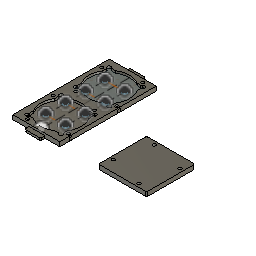
CoasterCutHolder_Double (Autodesk Fusion 360 design; units mm, degrees)
Autodesk Fusion 360 part; units mm, degrees
sketch "Sketch1" plane through (0, 0, 0) normal (0, 0, 1) x (1, 0, 0)
  line L0 (0, 0) -> (110, 0)
  line L1 (110, 0) -> (110, 110)
  line L2 (110, 110) -> (0, 110)
  line L3 (0, 110) -> (0, 0)
  line L4 (152.6101, 110) -> (152.6101, -10) construction
  line L5 (305.2202, 110) -> (305.2202, 0)
  line L6 (305.2202, 0) -> (195.2202, 0)
  line L7 (195.2202, 0) -> (195.2202, 110)
  line L8 (195.2202, 110) -> (305.2202, 110)
  line L9 (211.6202, 93.6) -> (288.8202, 93.6) construction
  line L10 (288.8202, 93.6) -> (288.8202, 16.4) construction
  line L11 (288.8202, 16.4) -> (211.6202, 16.4) construction
  line L12 (211.6202, 16.4) -> (211.6202, 93.6) construction
  line L13 (260, 93.6) -> (260, 110) construction
  line L14 (258.2734, 16.4) -> (258.2734, 0) construction
  line L15 (288.8202, 57.8839) -> (305.2202, 57.8839) construction
  line L16 (211.6202, 57.8839) -> (195.2202, 57.8839) construction
  line L17 (250.2202, 93.6) -> (250.2202, 110) construction
  line L18 (288.8202, 55) -> (305.2202, 55) construction
  line L19 (250.2202, 16.4) -> (250.2202, 0) construction
  line L20 (211.6202, 55) -> (195.2202, 55) construction
  line L21 (110, 67.7) -> (110, 42.3)
  line L22 (0, 42.3) -> (0, 67.7)
  line L23 (-12.7, 55) -> (0, 55) construction
  line L24 (0, 55) -> (110, 55) construction
  line L25 (122.7, 55) -> (110, 55) construction
  point P0 (250.2202, 8.2)
  point P1 (297.0202, 55)
  point P2 (250.2202, 101.8)
  point P3 (203.4202, 55)
  dimension "d3" = 110
  dimension "d4" = 110
  dimension "d17" = 77.2
  constraint horizontal L0
  constraint vertical L1
  constraint horizontal L2
  constraint vertical L3
  constraint coincident L0.start L3.end
  constraint vertical L4
  constraint symmetric L0.start L4 L5.end
  constraint symmetric L0.end L4 L6.end
  constraint symmetric L1.end L4 L7.end
  constraint symmetric L2.end L4 L5.start
  constraint horizontal L9
  constraint vertical L10
  constraint horizontal L11
  constraint vertical L12
  constraint coincident L9 L13.start
  constraint coincident L8 L13.end
  constraint perpendicular L8 L13
  constraint coincident L11 L14.start
  constraint coincident L6 L14.end
  constraint perpendicular L6 L14
  constraint coincident L10 L15.start
  constraint coincident L5 L15.end
  constraint perpendicular L5 L15
  constraint coincident L12 L16.start
  constraint coincident L7 L16.end
  constraint perpendicular L7 L16
  constraint equal L15 L16
  constraint equal L13 L15
  constraint equal L13 L14
  constraint midpoint L9 L17.start
  constraint midpoint L8 L17.end
  constraint midpoint L10 L18.start
  constraint midpoint L5 L18.end
  constraint midpoint L11 L19.start
  constraint midpoint L6 L19.end
  constraint midpoint L12 L20.start
  constraint midpoint L7 L20.end
  constraint midpoint L19 P0
  constraint midpoint L18 P1
  constraint midpoint L17 P2
  constraint midpoint L20 P3
  constraint vertical L21
  constraint coincident L1 L21.end
  constraint vertical L22
  constraint coincident L3 L22.end
  constraint midpoint L22 L23.end
  constraint midpoint L3 L23.end
  constraint midpoint L1 L24.end
  constraint midpoint L21 L24.end
  constraint collinear L23 L24
  measures "d3" distance of L0.start L2.end
  measures "d4" distance of L0.start L0.end
  measures "d17" distance of L9.start L9.end
extrude "Extrude1" add sketch "Sketch1" along normal blind 10 contours L0 L1 L2 L3 L21 L22 makes body 1
sketch "Sketch2" plane through (0, 0, 10) normal (0, 0, 1) x (-1, 0, 0)
  line L0 (0, -110) -> (0, 0)
  line L1 (0, 0) -> (-110, 0)
  line L2 (-110, 0) -> (-110, -110)
  line L3 (-110, -110) -> (0, -110)
  line L4 (-16.4, -93.6) -> (-93.6, -93.6)
  line L5 (-93.6, -93.6) -> (-93.6, -16.4)
  line L6 (-93.6, -16.4) -> (-16.4, -16.4)
  line L7 (-16.4, -16.4) -> (-16.4, -93.6)
  line L8 (0, -65.0851) -> (-16.4, -65.0851) construction
  line L9 (-93.6, -65.0851) -> (-110, -65.0851) construction
  line L10 (-60.9171, -93.6) -> (-60.9171, -110) construction
  line L11 (-67.2958, -16.4) -> (-67.2958, 0) construction
  circle A0 centre (-16.4, -93.6) radius 4
  circle A1 centre (-93.6, -93.6) radius 4
  circle A2 centre (-93.6, -16.4) radius 4
  circle A3 centre (-16.4, -16.4) radius 4
  line L12 (0, -84.4385) -> (-16.4, -84.0438) construction
  line L13 (-25.6464, -16.4) -> (-25.6464, 0) construction
  line L14 (-93.6, -25.6464) -> (-110, -25.6464) construction
  line L15 (-84.3536, -93.6) -> (-84.3536, -110) construction
  line L16 (-110, -110) -> (0, -110)
  line L17 (-110, 0) -> (-110, -110)
  line L18 (0, 0) -> (-110, 0)
  line L19 (0, -110) -> (0, 0)
  line L20 (-3.5294, -84.3536) -> (-3.5294, -110) construction
  line L21 (-84.3536, -105.8553) -> (-110, -105.8553) construction
  line L22 (-100.2693, -25.6464) -> (-100.2693, 0) construction
  line L23 (-25.6464, -11.6896) -> (0, -11.6896) construction
  line L24 (-152.6101, -110) -> (-152.6101, 10)
  circle A4 centre (-220.8667, -101.8) radius 3.7
  circle A5 centre (-297.0202, -84.2411) radius 3.7
  circle A6 centre (-279.5738, -8.2) radius 3.7
  circle A7 centre (-203.4202, -25.6464) radius 3.7
  line L25 (-94.1, -94.1) -> (-94.1, -15.9)
  line L26 (-94.1, -15.9) -> (-15.9, -15.9)
  line L27 (-15.9, -15.9) -> (-15.9, -94.1)
  line L28 (-15.9, -94.1) -> (-94.1, -94.1)
  line L29 (-81.6113, -96.8526) -> (-87.267, -96.9514)
  line L30 (-87.267, -96.9514) -> (-90.0093, -101.8989)
  line L31 (-90.0093, -101.8989) -> (-87.0958, -106.7474)
  line L32 (-87.0958, -106.7474) -> (-81.4401, -106.6486)
  line L33 (-81.4401, -106.6486) -> (-78.6978, -101.7011)
  line L34 (-78.6978, -101.7011) -> (-81.6113, -96.8526)
  line L35 (-13.0385, -80.7682) -> (-13.6269, -86.695)
  line L36 (-13.6269, -86.695) -> (-8.7884, -90.1679)
  line L37 (-8.7884, -90.1679) -> (-3.3615, -87.7141)
  line L38 (-3.3615, -87.7141) -> (-2.7731, -81.7873)
  line L39 (-2.7731, -81.7873) -> (-7.6116, -78.3144)
  line L40 (-7.6116, -78.3144) -> (-13.0385, -80.7682)
  line L41 (-28.1606, -3.9061) -> (-30.6222, -8.2304)
  line L42 (-30.6222, -8.2304) -> (-28.108, -12.5243)
  line L43 (-28.108, -12.5243) -> (-23.1323, -12.4939)
  line L44 (-23.1323, -12.4939) -> (-20.6707, -8.1696)
  line L45 (-20.6707, -8.1696) -> (-23.1849, -3.8757)
  line L46 (-23.1849, -3.8757) -> (-28.1606, -3.9061)
  line L47 (-99.3875, -21.5819) -> (-104.1138, -21.5248)
  line L48 (-104.1138, -21.5248) -> (-106.5263, -25.5894)
  line L49 (-106.5263, -25.5894) -> (-104.2125, -29.711)
  line L50 (-104.2125, -29.711) -> (-99.4862, -29.768)
  line L51 (-99.4862, -29.768) -> (-97.0737, -25.7035)
  line L52 (-97.0737, -25.7035) -> (-99.3875, -21.5819)
  point P0 (-8.2, -84.2411)
  point P1 (-84.3536, -101.8)
  point P2 (-101.8, -25.6464)
  point P3 (-25.6464, -8.2)
  point P4 (-220.8667, -101.8)
  point P5 (-297.0202, -84.2411)
  point P6 (-279.5738, -8.2)
  point P7 (-203.4202, -25.6464)
  point P8 (-84.3536, -101.8)
  point P9 (-8.2, -84.2411)
  point P10 (-25.6464, -8.2)
  point P11 (-101.8, -25.6464)
  dimension "d7" = 77.2
  dimension "d8" = 77.2
  dimension "d11" = 8
  dimension "d35" = 7.4
  dimension "d37" = -0.5
  constraint horizontal L4
  constraint vertical L5
  constraint horizontal L6
  constraint vertical L7
  constraint coincident L0 L8.start
  constraint coincident L7 L8.end
  constraint perpendicular L7 L8
  constraint coincident L5 L9.start
  constraint coincident L2 L9.end
  constraint perpendicular L2 L9
  constraint coincident L4 L10.start
  constraint coincident L3 L10.end
  constraint perpendicular L3 L10
  constraint coincident L6 L11.start
  constraint coincident L1 L11.end
  constraint perpendicular L1 L11
  constraint equal L10 L11
  constraint equal L8 L9
  constraint coincident L4.start L7.end
  constraint coincident L4.end L5.start
  constraint coincident L5.end L6.start
  constraint coincident L6.end L7.start
  constraint equal A0 A3
  constraint equal A0 A1
  constraint equal A1 A2
  constraint midpoint L12 P9
  constraint midpoint L15 P8
  constraint midpoint L14 P11
  constraint midpoint L13 P10
  constraint vertical L15
  constraint coincident L15.end L16
  constraint coincident L4 L15.start
  constraint coincident L14.end L17
  constraint coincident L5 L14.start
  constraint perpendicular L6 L13
  constraint coincident L13.end L18
  constraint coincident L6 L13.start
  constraint coincident L7 L12.end
  constraint coincident L12.start L19
  constraint coincident L12 L20.start
  constraint coincident L16 L20.end
  constraint perpendicular L16 L20
  constraint coincident L15 L21.start
  constraint coincident L17 L21.end
  constraint perpendicular L17 L21
  constraint coincident L14 L22.start
  constraint coincident L18 L22.end
  constraint perpendicular L18 L22
  constraint coincident L13 L23.start
  constraint coincident L19 L23.end
  constraint perpendicular L19 L23
  constraint equal L20 L21
  constraint equal L21 L22
  constraint equal L22 L23
  constraint symmetric P9 L24 P5
  constraint symmetric P8 L24 P4
  constraint symmetric P11 L24 P7
  constraint symmetric P10 L24 P6
  constraint coincident P4 A4.centre
  constraint coincident P5 A5.centre
  constraint coincident P6 A6.centre
  constraint coincident P7 A7.centre
  constraint equal A4 A7
  constraint equal A4 A5
  constraint equal A5 A6
  constraint coincident P8 P1
  constraint coincident P9 P0
  constraint coincident P10 P3
  constraint coincident P11 P2
  constraint horizontal L14
  measures "d7" distance of L4.end L5.end
  measures "d8" distance of L5.end L6.end
  measures "d11" diameter of A0
  measures "d35" diameter of A6
extrude "Extrude2" cut sketch "Sketch2" against normal blind 5 contours L4 L5 A1 L25 L28 | L4 L5 L6 L7 A0 A1 A2 A3 | L4 L5 A1 | L4 A0 A1 L28 | L4 L7 A0 | L4 L7 A0 L27 L28 | L5 A1 A2 L25 | A1 L25 L28 | L7 A0 A3 L27 | A0 L27 L28 | L5 L6 A2 L25 L26 | L5 L6 A2 | L6 L7 A3 | L6 L7 A3 L26 L27 | A2 L25 L26 | L6 A2 A3 L26 | A3 L26 L27 bodies 1
hole "Hole1" at (8.2, 84.2411, 10) at (25.6464, 8.2, 10) at (84.3536, 101.8, 10) at (101.8, 25.6464, 10) direction (0, 0, -1) diameter 7 depth 10 tip angle 118 bodies 1
extrude "Extrude3" add sketch "Sketch1" along normal blind 10 separate body contours L5 L6 L7 L8 makes body 2
fillet "Fillet2" radius 3 4 edges at (195.2202, 0, 5) (305.2202, 0, 5) (305.2202, 110, 5) (195.2202, 110, 5) on bodies 2
fillet "Fillet3" radius 2 8 edges at (89.6314, 15.9, 7.5) (94.1, 20.3686, 7.5) (94.1, 89.6314, 7.5) (89.6314, 94.1, 7.5) (20.3686, 94.1, 7.5) (15.9, 89.6314, 7.5) (15.9, 20.3686, 7.5) (20.3686, 15.9, 7.5) on bodies 1
sketch "Sketch5" plane through (0, 0, 5) normal (0, 0, 1) x (-1, 0, 0)
  arc A0 (-89.9638, -14.7333) -> (-95.2667, -20.0362) centre (-93.6, -16.4) ccw
  arc A1 (-95.2667, -89.9638) -> (-89.9638, -95.2667) centre (-93.6, -93.6) ccw
  arc A2 (-20.0362, -95.2667) -> (-14.7333, -89.9638) centre (-16.4, -93.6) ccw
  arc A3 (-14.7333, -20.0362) -> (-20.0362, -14.7333) centre (-16.4, -16.4) ccw
  line L0 (-16.4, -55) -> (-93.6, -55) construction
  line L1 (-55, -16.4) -> (-55, -93.6) construction
  circle A4 centre (-55, -55) radius 46.1041
  line L2 (-88.1456, -94.1) -> (-21.8544, -94.1)
  line L3 (-15.9, -88.1456) -> (-15.9, -21.8544)
  line L4 (-21.8544, -15.9) -> (-88.1456, -15.9)
  line L5 (-94.1, -21.8544) -> (-94.1, -88.1456)
  arc A5 (-89.9638, -14.7333) -> (-88.1456, -15.9) centre (-88.1456, -13.9) ccw
  arc A6 (-94.1, -21.8544) -> (-95.2667, -20.0362) centre (-96.1, -21.8544) ccw
  arc A7 (-95.2667, -89.9638) -> (-94.1, -88.1456) centre (-96.1, -88.1456) ccw
  arc A8 (-88.1456, -94.1) -> (-89.9638, -95.2667) centre (-88.1456, -96.1) ccw
  arc A9 (-20.0362, -95.2667) -> (-21.8544, -94.1) centre (-21.8544, -96.1) ccw
  arc A10 (-15.9, -88.1456) -> (-14.7333, -89.9638) centre (-13.9, -88.1456) ccw
  arc A11 (-14.7333, -20.0362) -> (-15.9, -21.8544) centre (-13.9, -21.8544) ccw
  arc A12 (-21.8544, -15.9) -> (-20.0362, -14.7333) centre (-21.8544, -13.9) ccw
  constraint vertical L1
  constraint midpoint L0 A4.centre
extrude "Extrude5" cut sketch "Sketch5" along normal up to surface (5 mm away) contours A4 L2 L3 L4 L5 | A4 L4 | A4 L5 | A4 L3 | A4 L2 bodies 1
extrude "Extrude6" cut sketch "Sketch2" against normal through all contours A4 | A5 | A6 | A7 bodies 2
pattern_linear "R-Pattern1" count 2 spacing 110 along (0, 1, 0) of bodies 1 makes body 3
sketch "Sketch6" plane through (0, 0, 0) normal (0, 0, -1) x (1, 0, 0)
  line L0 (0, -110) -> (0, -220)
  line L1 (0, -220) -> (110, -220)
  line L2 (110, -220) -> (110, -110)
  line L3 (110, -110) -> (0, -110)
  line L4 (72.9884, -220) -> (37.0116, -220)
  line L5 (37.0116, -220) -> (37.0116, -230)
  line L6 (37.0116, -230) -> (72.9884, -230)
  line L7 (72.9884, -230) -> (72.9884, -220)
  line L8 (72.9884, 0) -> (37.0116, 0)
  line L9 (37.0116, 0) -> (37.0116, 10)
  line L10 (37.0116, 10) -> (72.9884, 10)
  line L11 (72.9884, 10) -> (72.9884, 0)
  line L12 (0, 0) -> (110, 0)
  line L13 (55, -55) -> (55, -230) construction
  line L14 (55, -55) -> (55, 10) construction
  circle A0 centre (84.3536, -211.8) radius 3.5
  circle A1 centre (8.2, -194.2411) radius 3.5
  circle A2 centre (25.6464, -118.2) radius 3.5
  circle A3 centre (101.8, -135.6464) radius 3.5
  point P0 (55, -55)
  dimension "d44" = 10
  constraint horizontal L4
  constraint vertical L5
  constraint horizontal L6
  constraint vertical L7
  constraint coincident L1 L4.start
  constraint horizontal L8
  constraint vertical L9
  constraint horizontal L10
  constraint vertical L11
  constraint equal L5 L9
  constraint collinear L8 L12
  constraint midpoint L6 L13.end
  constraint vertical L13
  constraint coincident P0 L13.start
  constraint midpoint L10 L14.end
  constraint vertical L14
  measures "d44" distance of L4.end L5.end
extrude "Extrude7" add sketch "Sketch6" against normal blind 5 contours L1 L4 L5 L6 L7 | L8 L9 L10 L11 L12 bodies 1 3
fillet "Fillet4" radius 3 4 edges at (37.0116, -10, 2.5) (72.9884, -10, 2.5) (37.0116, 230, 2.5) (72.9884, 230, 2.5) on bodies 1 3
sketch "Sketch7" plane through (0, 0, 0) normal (0, 0, -1) x (1, 0, 0)
  arc A0 (69.9884, -230) -> (72.9884, -227) centre (69.9884, -227) ccw
  line L0 (72.9884, -227) -> (72.9884, -220)
  line L1 (72.9884, -220) -> (110, -220)
  line L2 (110, -220) -> (110, -110)
  line L3 (110, -110) -> (0, -110)
  line L4 (0, -110) -> (0, -220)
  line L5 (0, -220) -> (37.0116, -220)
  line L6 (37.0116, -220) -> (37.0116, -227)
  arc A1 (37.0116, -227) -> (40.0116, -230) centre (40.0116, -227) ccw
  line L7 (40.0116, -230) -> (69.9884, -230)
  line L8 (80.0822, -208.841) -> (79.6553, -214.0196)
  line L9 (79.6553, -214.0196) -> (83.9266, -216.9786)
  line L10 (83.9266, -216.9786) -> (88.6249, -214.759)
  line L11 (88.6249, -214.759) -> (89.0518, -209.5804)
  line L12 (89.0518, -209.5804) -> (84.7805, -206.6214)
  line L13 (84.7805, -206.6214) -> (80.0822, -208.841)
  line L14 (7.4239, -189.1033) -> (3.3624, -192.3443)
  line L15 (3.3624, -192.3443) -> (4.1385, -197.4822)
  line L16 (4.1385, -197.4822) -> (8.9761, -199.379)
  line L17 (8.9761, -199.379) -> (13.0376, -196.138)
  line L18 (13.0376, -196.138) -> (12.2615, -191.0001)
  line L19 (12.2615, -191.0001) -> (7.4239, -189.1033)
  line L20 (97.3066, -138.2559) -> (101.8132, -140.8426)
  line L21 (101.8132, -140.8426) -> (106.3066, -138.2331)
  line L22 (106.3066, -138.2331) -> (106.2934, -133.037)
  line L23 (106.2934, -133.037) -> (101.7868, -130.4503)
  line L24 (101.7868, -130.4503) -> (97.2934, -133.0598)
  line L25 (97.2934, -133.0598) -> (97.3066, -138.2559)
  line L26 (30.8086, -117.6064) -> (27.7134, -113.4327)
  line L27 (27.7134, -113.4327) -> (22.5513, -114.0263)
  line L28 (22.5513, -114.0263) -> (20.4843, -118.7936)
  line L29 (20.4843, -118.7936) -> (23.5794, -122.9673)
  line L30 (23.5794, -122.9673) -> (28.7416, -122.3737)
  line L31 (28.7416, -122.3737) -> (30.8086, -117.6064)
  circle A2 centre (84.3536, -211.8) radius 3.5
  circle A3 centre (8.2, -194.2411) radius 3.5
  circle A4 centre (25.6464, -118.2) radius 3.5
  circle A5 centre (101.8, -135.6464) radius 3.5
  point P0 (84.3536, -211.8)
  point P1 (8.2, -194.2411)
  point P2 (101.8, -135.6464)
  point P3 (25.6464, -118.2)
  dimension "d49" = 9
  constraint coincident P0 A2.centre
  constraint coincident P1 A3.centre
  constraint coincident P2 A5.centre
  constraint coincident P3 A4.centre
  constraint equal L24 L26
  constraint equal L18 L25
  constraint equal L8 L18
  measures "d49" distance of L15 L18
extrude "Extrude8" cut sketch "Sketch7" against normal blind 6 contours L8 L9 L10 L11 L12 L13 | L14 L15 L16 L17 L18 L19 | L20 L21 L22 L23 L24 L25 | L26 L27 L28 L29 L30 L31 | A2 | A3 | A4 | A5 bodies 3
sketch "Sketch11" plane through (0, 0, 0) normal (0, 0, -1) x (1, 0, 0)
  arc A0 (72.9884, 7) -> (69.9884, 10) centre (69.9884, 7) ccw
  line L0 (69.9884, 10) -> (40.0116, 10)
  arc A1 (40.0116, 10) -> (37.0116, 7) centre (40.0116, 7) ccw
  line L1 (37.0116, 7) -> (37.0116, 0)
  line L2 (37.0116, 0) -> (0, 0)
  line L3 (0, 0) -> (0, -110)
  line L4 (0, -110) -> (110, -110)
  line L5 (110, -110) -> (110, 0)
  line L6 (110, 0) -> (72.9884, 0)
  line L7 (72.9884, 0) -> (72.9884, 7)
  line L8 (30.1482, -10.7951) -> (30.1447, -5.5989)
  line L9 (30.1447, -5.5989) -> (25.643, -3.0038)
  line L10 (25.643, -3.0038) -> (21.1447, -5.6049)
  line L11 (21.1447, -5.6049) -> (21.1482, -10.8011)
  line L12 (21.1482, -10.8011) -> (25.6499, -13.3962)
  line L13 (25.6499, -13.3962) -> (30.1482, -10.7951)
  line L14 (7.7111, -79.068) -> (3.4755, -82.078)
  line L15 (3.4755, -82.078) -> (3.9644, -87.2511)
  line L16 (3.9644, -87.2511) -> (8.6889, -89.4142)
  line L17 (8.6889, -89.4142) -> (12.9245, -86.4043)
  line L18 (12.9245, -86.4043) -> (12.4356, -81.2312)
  line L19 (12.4356, -81.2312) -> (7.7111, -79.068)
  line L20 (97.2154, -28.0921) -> (101.6257, -30.8397)
  line L21 (101.6257, -30.8397) -> (106.2103, -28.394)
  line L22 (106.2103, -28.394) -> (106.3846, -23.2008)
  line L23 (106.3846, -23.2008) -> (101.9743, -20.4532)
  line L24 (101.9743, -20.4532) -> (97.3897, -22.8989)
  line L25 (97.3897, -22.8989) -> (97.2154, -28.0921)
  line L26 (81.7555, -97.3) -> (79.1574, -101.8)
  line L27 (79.1574, -101.8) -> (81.7555, -106.3)
  line L28 (81.7555, -106.3) -> (86.9516, -106.3)
  line L29 (86.9516, -106.3) -> (89.5497, -101.8)
  line L30 (89.5497, -101.8) -> (86.9516, -97.3)
  line L31 (86.9516, -97.3) -> (81.7555, -97.3)
  circle A2 centre (84.3536, -101.8) radius 3.5
  circle A3 centre (8.2, -84.2411) radius 3.5
  circle A4 centre (25.6464, -8.2) radius 3.5
  circle A5 centre (101.8, -25.6464) radius 3.5
  point P0 (25.6464, -8.2)
  point P1 (8.2, -84.2411)
  point P2 (101.8, -25.6464)
  point P3 (84.3536, -101.8)
  dimension "d54" = 9
  constraint coincident P0 A4.centre
  constraint coincident P1 A3.centre
  constraint coincident P2 A5.centre
  constraint coincident P3 A2.centre
  constraint equal L18 L30
  constraint equal L18 L25
  constraint equal L9 L24
  measures "d54" distance of L28 L31
extrude "Extrude10" cut sketch "Sketch11" against normal blind 6 contours L8 L9 L10 L11 L12 L13 | L14 L15 L16 L17 L18 L19 | L20 L21 L22 L23 L24 L25 | L26 L27 L28 L29 L30 L31 | A2 | A3 | A4 | A5 bodies 1
combine "Combine1" operation add target body 1 tool bodies 3
sketch "Sketch12" plane through (0, 0, 5) normal (0, 0, 1) x (-1, 0, 0)
  line L0 (-79.429, -125.9) -> (-88.1456, -125.9)
  arc A0 (-89.9638, -124.7333) -> (-88.1456, -125.9) centre (-88.1456, -123.9) ccw
  arc A1 (-89.9638, -124.7333) -> (-95.2667, -130.0362) centre (-93.6, -126.4) ccw
  arc A2 (-94.1, -131.8544) -> (-95.2667, -130.0362) centre (-96.1, -131.8544) ccw
  line L1 (-94.1, -131.8544) -> (-94.1, -140.571)
  arc A3 (-94.1, -140.571) -> (-94.1, -189.429) centre (-55, -165) ccw
  line L2 (-94.1, -189.429) -> (-94.1, -198.1456)
  arc A4 (-95.2667, -199.9638) -> (-94.1, -198.1456) centre (-96.1, -198.1456) ccw
  arc A5 (-95.2667, -199.9638) -> (-89.9638, -205.2667) centre (-93.6, -203.6) ccw
  arc A6 (-88.1456, -204.1) -> (-89.9638, -205.2667) centre (-88.1456, -206.1) ccw
  line L3 (-88.1456, -204.1) -> (-79.429, -204.1)
  arc A7 (-79.429, -204.1) -> (-30.571, -204.1) centre (-55, -165) ccw
  line L4 (-30.571, -204.1) -> (-21.8544, -204.1)
  arc A8 (-20.0362, -205.2667) -> (-21.8544, -204.1) centre (-21.8544, -206.1) ccw
  arc A9 (-20.0362, -205.2667) -> (-14.7333, -199.9638) centre (-16.4, -203.6) ccw
  arc A10 (-15.9, -198.1456) -> (-14.7333, -199.9638) centre (-13.9, -198.1456) ccw
  line L5 (-15.9, -198.1456) -> (-15.9, -189.429)
  arc A11 (-15.9, -189.429) -> (-15.9, -140.571) centre (-55, -165) ccw
  line L6 (-15.9, -140.571) -> (-15.9, -131.8544)
  arc A12 (-14.7333, -130.0362) -> (-15.9, -131.8544) centre (-13.9, -131.8544) ccw
  arc A13 (-14.7333, -130.0362) -> (-20.0362, -124.7333) centre (-16.4, -126.4) ccw
  arc A14 (-21.8544, -125.9) -> (-20.0362, -124.7333) centre (-21.8544, -123.9) ccw
  line L7 (-21.8544, -125.9) -> (-30.571, -125.9)
  arc A15 (-30.571, -125.9) -> (-79.429, -125.9) centre (-55, -165) ccw
  line L8 (-55, -211.1041) -> (-55, -10) construction
  line L9 (-55, -177.6615) -> (-77.5, -177.6615) construction
  line L10 (-55, -177.6615) -> (-32.5, -177.6615) construction
  line L11 (-32.5, -177.6615) -> (-32.5, -132.6615) construction
  line L12 (-32.5, -132.6615) -> (-77.5, -132.6615) construction
  line L13 (-77.5, -132.6615) -> (-77.5, -177.6615) construction
  line L14 (-32.5, -132.6615) -> (-32.5, -87.6615) construction
  line L15 (-32.5, -87.6615) -> (-77.5, -87.6615) construction
  line L16 (-77.5, -87.6615) -> (-77.5, -132.6615) construction
  line L17 (-32.5, -87.6615) -> (-32.5, -42.6615) construction
  line L18 (-32.5, -42.6615) -> (-77.5, -42.6615) construction
  line L19 (-77.5, -42.6615) -> (-77.5, -87.6615) construction
  circle A16 centre (-32.5, -177.6615) radius 5.25
  circle A17 centre (-77.5, -177.6615) radius 5.25
  circle A18 centre (-77.5, -132.6615) radius 5.25
  circle A19 centre (-32.5, -132.6615) radius 5.25
  circle A20 centre (-32.5, -87.6615) radius 5.25
  circle A21 centre (-77.5, -87.6615) radius 5.25
  circle A22 centre (-77.5, -42.6615) radius 5.25
  circle A23 centre (-32.5, -42.6615) radius 5.25
  circle A24 centre (-32.5, -42.6615) radius 3
  circle A25 centre (-77.5, -42.6615) radius 3
  circle A26 centre (-77.5, -87.6615) radius 3
  circle A27 centre (-32.5, -87.6615) radius 3
  circle A28 centre (-32.5, -132.6615) radius 3
  circle A29 centre (-77.5, -132.6615) radius 3
  circle A30 centre (-77.5, -177.6615) radius 3
  circle A31 centre (-32.5, -177.6615) radius 3
  dimension "d57" = 45
  dimension "d58" = 45
  dimension "d59" = 45
  dimension "d60" = 45
  dimension "d61" = 10.5
  dimension "d64" = 6
  constraint midpoint A7 L8.start
  constraint vertical L8
  constraint coincident L8 L9.start
  constraint perpendicular L8 L9
  constraint perpendicular L8 L10
  constraint equal L9 L10
  constraint perpendicular L10 L11
  constraint perpendicular L8 L12
  constraint vertical L13
  constraint perpendicular L12 L14
  constraint perpendicular L8 L15
  constraint vertical L16
  constraint perpendicular L15 L17
  constraint vertical L19
  constraint horizontal L18
  constraint coincident L10.end L11.start
  constraint coincident L9.end L13.end
  constraint coincident L12.end L13.start
  constraint coincident L11.end L12.start
  constraint coincident L14.end L15.start
  constraint coincident L15.end L16.start
  constraint coincident L18.end L19.start
  constraint coincident L17.end L18.start
  constraint equal A16 A17
  constraint equal A17 A18
  constraint equal A18 A19
  constraint equal A19 A20
  constraint equal A20 A21
  constraint equal A21 A22
  constraint equal A22 A23
  constraint concentric A23 A24
  constraint concentric A22 A25
  constraint concentric A21 A26
  constraint concentric A20 A27
  constraint equal A26 A27
  constraint equal A24 A25
  constraint concentric A19 A28
  constraint concentric A18 A29
  constraint concentric A17 A30
  constraint concentric A16 A31
  constraint equal A30 A31
  constraint equal A29 A30
  constraint equal A28 A29
  constraint equal A27 A28
  constraint equal A25 A26
  measures "d57" distance of L9.end L10.end
  measures "d58" distance of L10.end L11.end
  measures "d59" distance of L12.end L15.end
  measures "d60" distance of L15.end L18.end
  measures "d61" diameter of A17
  measures "d64" diameter of A31
extrude "Extrude11" cut sketch "Sketch12" against normal blind 2 contours A16 | A17 | A18 | A19 | A20 | A21 | A22 | A23 | A24 | A25 | A26 | A27 | A28 | A29 | A30 | A31 bodies 1
extrude "Extrude12" cut sketch "Sketch12" against normal up to surface (5 mm away) contours A24 | A25 | A26 | A27 | A28 | A29 | A30 | A31 bodies 1
extrude "Extrude13" cut 1 faces at (110, 73.3333, 3.3333) along direction (-1, 0, 0) blind 3 on bodies 1 bodies 1
equation "wPocket = 3 * 25.4 mm + 1 mm"
equation "wOuter = 110 mm"
equation "d3 = wOuter"
equation "d4 = wOuter"
equation "d7 = wPocket"
equation "d8 = wPocket"
equation "d17 = wPocket"
